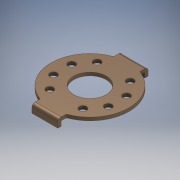
# Autodesk Inventor part: SŁONECZKO MAŁE
Saved by Autodesk Inventor 2017 SP1 (Build 210196100, 196)
## iProperties
Created: 2021-02-08
Part Number: SŁONECZKO MAŁE
Material: Stal
Document SubType Name: Modeling
Designer: Napoleon
Mass: 0.390645 g
Surface Area: 2.43287 cm^2
Volume: 0.0497637 cm^3
Density: 7.85 g/cm^3
Appearance: Anodowany - brązowy
Author: Napoleon
Autodesk Inventor part; units mm, degrees
ref_plane "YZ Plane" through (0, 0, 0) normal (1, 0, 0) x (0, 1, 0)
ref_plane "XZ Plane" through (0, 0, 0) normal (0, 1, 0) x (-1, 0, 0)
ref_plane "XY Plane" through (0, 0, 0) normal (0, 0, 1) x (1, 0, 0)
sketch "Szkic1" plane through (0, 0, 0) normal (0, 0, 1) x (1, 0, 0)
  circle A0 centre (0, 0) radius 2.5
  line L0 (-2, 6.95) -> (2, 6.95)
  line L1 (-2, -6.95) -> (2, -6.95)
  line L2 (-2, 6.95) -> (-2, 5.6569)
  line L3 (2, 6.95) -> (2, 5.6569)
  line L4 (-2, -6.95) -> (-2, -5.6569)
  line L5 (2, -6.95) -> (2, -5.6569)
  arc A1 (-2, 5.6569) -> (-2, -5.6569) centre (0, 0) ccw
  arc A2 (2, -5.6569) -> (2, 5.6569) centre (0, 0) ccw
  circle A3 centre (2.55, 3.6469) radius 0.55
  circle A4 centre (4.2238, 1.4007) radius 0.55
  circle A5 centre (4.2238, -1.4006) radius 0.55
  circle A6 centre (2.55, -3.6469) radius 0.55
  circle A7 centre (-2.55, 3.6469) radius 0.55
  circle A8 centre (-4.2238, 1.4007) radius 0.55
  circle A9 centre (-4.2238, -1.4006) radius 0.55
  circle A10 centre (-2.55, -3.6469) radius 0.55
  dimension "d4" = 4
  dimension "d5" = 4
  dimension "d25" = 110.076
  constraints: 12 end point, 11 centre point, 4 point on circle, 4 vertical, 2 horizontal, 1 coincident, 7 other
  measures "d4" distance of L0.start L0.end
  measures "d5" distance of L1.start L1.end
extrude "Wyciągnięcie proste3" add sketch "Szkic1" against normal blind 0.5
sketch "Szkic3" plane through (0, 0, -0.5) normal (0, 0, -1) x (-1, 0, 0)
  line L0 (2, 6.95) -> (-2, 6.95) projected
  line L1 (-2, 6.95) -> (2, 6.95)
  line L2 (2, 6.95) -> (2, 6.45)
  line L3 (2, 6.45) -> (-2, 6.45)
  line L4 (-2, 6.45) -> (-2, 6.95)
  line L5 (-2, -6.95) -> (2, -6.95) projected
  line L6 (-2, -6.95) -> (2, -6.95)
  line L7 (2, -6.95) -> (2, -6.45)
  line L8 (2, -6.45) -> (-2, -6.45)
  line L9 (-2, -6.45) -> (-2, -6.95)
  constraints: 16 end point, 4 parallel, 2 horizontal, 2 perpendicular
extrude "Wyciągnięcie proste4" add sketch "Szkic3" along normal blind 0.75
fillet "Zaokrąglenie3" radius 0.25 4 edges at (-2, 5.6569, -0.25) (2, 5.6569, -0.25) (2, -5.6569, -0.25) (-2, -5.6569, -0.25)
fillet "Zaokrąglenie4" radius 0.5 2 edges at (0, -6.95, 0) (0, 6.95, 0)
